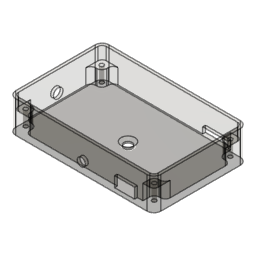
LCD Box (Autodesk Fusion 360 design; units mm, degrees)
Autodesk Fusion 360 part; units mm, degrees
sketch "Sketch1" plane through (0, 0, 0) normal (0, 1, 0) x (1, 0, 0)
  line L0 (-52.5, 33.75) -> (52.5, 33.75)
  line L1 (52.5, 33.75) -> (52.5, -33.75)
  line L2 (52.5, -33.75) -> (-52.5, -33.75)
  line L3 (-52.5, -33.75) -> (-52.5, 33.75)
  line L4 (-52.5, 33.75) -> (52.5, -33.75) construction
  dimension "d1" = 105
  dimension "d2" = 67.5
  constraint horizontal L0
  constraint vertical L1
  constraint horizontal L2
  constraint vertical L3
  constraint midpoint origin L4
  measures "d1" distance of L0.start L0.end
  measures "d2" distance of L0.start L2.end
extrude "Extrude1" add sketch "Sketch1" along normal blind 3
sketch "Sketch2" plane through (0, 3, 0) normal (0, 1, 0) x (-1, 0, 0)
  line L0 (52.5, 33.75) -> (-52.5, 33.75)
  line L1 (-52.5, 33.75) -> (-52.5, -33.75)
  line L2 (-52.5, -33.75) -> (52.5, -33.75)
  line L3 (52.5, -33.75) -> (52.5, 33.75)
  line L4 (50.5, 31.75) -> (-50.5, 31.75)
  line L5 (-50.5, 31.75) -> (-50.5, -31.75)
  line L6 (-50.5, -31.75) -> (50.5, -31.75)
  line L7 (50.5, -31.75) -> (50.5, 31.75)
  dimension "d5" = -2
extrude "Extrude2" add sketch "Sketch2" along normal blind 20
sketch "Sketch3" plane through (0, 0, -33.75) normal (0, 0, -1) x (-1, 0, 0)
  line L0 (-52.5, 0) -> (52.5, 0)
  line L1 (52.5, 0) -> (52.5, 23)
  line L2 (52.5, 23) -> (-52.5, 23)
  line L3 (-52.5, 23) -> (-52.5, 0)
  line L4 (-40.5, 7.5) -> (-22.25, 7.5)
  line L5 (-22.25, 7.5) -> (-22.25, 3)
  line L6 (-22.25, 3) -> (-40.5, 3)
  line L7 (-40.5, 3) -> (-40.5, 7.5)
  dimension "d21" = 18.25
  dimension "d22" = 4.5
  dimension "d23" = 3
  dimension "d24" = 40.5
  constraint horizontal L4
  constraint vertical L5
  constraint horizontal L6
  constraint vertical L7
  measures "d21" distance of L5.end L6.end
  measures "d22" distance of L4.start L6.end
  measures "d23" distance of origin L6
  measures "d24" distance of origin L7
extrude "Extrude3" cut sketch "Sketch3" against normal blind 3 contours L4 L5 L6 L7
sketch "Sketch4" plane through (0, 3, 0) normal (0, 1, 0) x (-1, 0, 0)
  line L0 (-22.25, -31.75) -> (50.5, -31.75)
  line L1 (50.5, -31.75) -> (50.5, 31.75)
  line L2 (50.5, 31.75) -> (-50.5, 31.75)
  line L3 (-50.5, 31.75) -> (-50.5, -31.75)
  line L4 (-50.5, -31.75) -> (-40.5, -31.75)
  line L5 (-40.5, -31.75) -> (-40.5, -33.75)
  line L6 (-40.5, -33.75) -> (-22.25, -33.75)
  line L7 (-22.25, -33.75) -> (-22.25, -31.75)
  line L8 (46.5, -27.5) -> (-46.5, -27.5) construction
  line L9 (-46.5, -27.5) -> (-46.5, 27.5) construction
  line L10 (-46.5, 27.5) -> (46.5, 27.5) construction
  line L11 (46.5, 27.5) -> (46.5, -27.5) construction
  line L12 (46.5, -27.5) -> (-46.5, 27.5) construction
  circle A0 centre (46.5, -27.5) radius 1.5
  line L13 (50.5, -23.5) -> (42.5, -23.5)
  line L14 (42.5, -23.5) -> (42.5, -31.75)
  line L15 (50.5, 0) -> (-50.5, 0) construction
  line L16 (50.5, 23.5) -> (42.5, 23.5)
  line L17 (42.5, 23.5) -> (42.5, 31.75)
  circle A1 centre (46.5, 27.5) radius 1.5
  line L18 (0, -27.5) -> (0, 27.5) construction
  line L19 (-42.5, -23.5) -> (-42.5, -31.75)
  line L20 (-50.5, -23.5) -> (-42.5, -23.5)
  circle A2 centre (-46.5, -27.5) radius 1.5
  circle A3 centre (-46.5, 27.5) radius 1.5
  line L21 (-50.5, 23.5) -> (-42.5, 23.5)
  line L22 (-42.5, 23.5) -> (-42.5, 31.75)
  dimension "d33" = 93
  dimension "d34" = 55
  dimension "d35" = 3
  dimension "d36" = 4
  dimension "d37" = 4
  constraint horizontal L8
  constraint vertical L9
  constraint horizontal L10
  constraint vertical L11
  constraint midpoint origin L12
  constraint coincident L8.start L11.end
  constraint coincident L1 L13.start
  constraint perpendicular L1 L13
  constraint coincident L0 L14.end
  constraint perpendicular L0 L14
  constraint midpoint L1 L15.start
  constraint midpoint L3 L15.end
  constraint symmetric A0 L15 A1
  constraint symmetric L13.start L15 L16.start
  constraint symmetric L13.end L15 L16.end
  constraint symmetric L14.end L15 L17.end
  constraint midpoint L8 L18.start
  constraint midpoint L10 L18.end
  constraint symmetric A0 L18 A2
  constraint symmetric L13.start L18 L20.start
  constraint symmetric L13.end L18 L19.start
  constraint symmetric L14.end L18 L19.end
  constraint symmetric L16.start L18 L21.start
  constraint symmetric L16.end L18 L21.end
  constraint symmetric L17.end L18 L22.end
  constraint symmetric A1 L18 A3
  measures "d33" distance of L8.start L8.end
  measures "d34" distance of L8.start L10.end
  measures "d35" diameter of A0
  measures "d36" distance of L8.start L13
  measures "d37" distance of L8.start L14
extrude "Extrude4" add sketch "Sketch4" along normal blind 11 contours L0 L1 L13 L14 | L1 L2 L16 L17 | L3 L4 L19 L20 | L2 L3 L21 L22
fillet "Fillet1" radius 3 4 edges at (-50.5, 18.5, -31.75) (50.5, 18.5, -31.75) (50.5, 18.5, 31.75) (-50.5, 18.5, 31.75)
fillet "Fillet2" radius 5 4 edges at (-52.5, 11.5, 33.75) (52.5, 11.5, 33.75) (52.5, 11.5, -33.75) (-52.5, 11.5, -33.75)
sketch "Sketch5" plane through (0, 0, 33.75) normal (0, 0, 1) x (1, 0, 0)
  line L0 (47.5, 0) -> (47.5, 23)
  line L1 (47.5, 23) -> (-47.5, 23)
  line L2 (-47.5, 23) -> (-47.5, 0)
  line L3 (-47.5, 0) -> (47.5, 0)
  circle A0 centre (0, 7) radius 3
  line L4 (0, 7) -> (0, 0) construction
  dimension "d58" = 6
  dimension "d59" = 7
  constraint coincident A0.centre L4.start
  constraint coincident L4.end origin
  constraint vertical L4
  measures "d58" diameter of A0
  measures "d59" distance of A0.centre L4.end
extrude "Extrude5" cut sketch "Sketch5" against normal blind 3 contours A0
sketch "Sketch6" plane through (0, 0, 33.75) normal (0, 0, 1) x (1, 0, 0)
  circle A0 centre (0, 7) radius 3
  line L0 (47.5, 0) -> (47.5, 23)
  line L1 (47.5, 23) -> (-47.5, 23)
  line L2 (-47.5, 23) -> (-47.5, 0)
  line L3 (-47.5, 0) -> (47.5, 0)
  line L4 (24, 10.5) -> (38.5, 10.5)
  line L5 (38.5, 10.5) -> (38.5, 3)
  line L6 (38.5, 3) -> (24, 3)
  line L7 (24, 3) -> (24, 10.5)
  dimension "d62" = 3
  dimension "d63" = 24
  dimension "d64" = 14.5
  dimension "d65" = 7.5
  constraint horizontal L4
  constraint vertical L5
  constraint horizontal L6
  constraint vertical L7
  measures "d62" distance of origin L6
  measures "d63" distance of origin L7
  measures "d64" distance of L4.start L4.end
  measures "d65" distance of L4.end L5.end
extrude "Extrude6" cut sketch "Sketch6" against normal blind 2 contours L4 L5 L6 L7
sketch "Sketch8" plane through (0, 3, 0) normal (0, 1, 0) x (-1, 0, 0)
  line L0 (-50.5, -23.5) -> (-42.5, -23.5)
  line L1 (-42.5, -23.5) -> (-42.5, -31.75)
  line L2 (-42.5, -31.75) -> (-40.5, -31.75)
  line L3 (-40.5, -31.75) -> (-40.5, -33.75)
  line L4 (-40.5, -33.75) -> (-22.25, -33.75)
  line L5 (-22.25, -33.75) -> (-22.25, -31.75)
  line L6 (-22.25, -31.75) -> (42.5, -31.75)
  line L7 (42.5, -31.75) -> (42.5, -23.5)
  line L8 (42.5, -23.5) -> (50.5, -23.5)
  line L9 (50.5, -23.5) -> (50.5, 23.5)
  line L10 (50.5, 23.5) -> (42.5, 23.5)
  line L11 (42.5, 23.5) -> (42.5, 31.75)
  line L12 (42.5, 31.75) -> (-24, 31.75)
  line L13 (-24, 31.75) -> (-24, 33.75)
  line L14 (-24, 33.75) -> (-38.5, 33.75)
  line L15 (-38.5, 33.75) -> (-38.5, 31.75)
  line L16 (-38.5, 31.75) -> (-42.5, 31.75)
  line L17 (-42.5, 31.75) -> (-42.5, 23.5)
  line L18 (-42.5, 23.5) -> (-50.5, 23.5)
  line L19 (-50.5, 23.5) -> (-50.5, -23.5)
  circle A0 centre (0, 0) radius 3
  dimension "d73" = 6
  constraint coincident A0.centre origin
  measures "d73" diameter of A0
extrude "Extrude8" cut sketch "Sketch8" against normal blind 6 contours A0
chamfer "Chamfer1" distance 2 angle 45 1 edges at (2.797, 3, 1.0848)
sketch "Sketch9" plane through (-52.5, 0, 0) normal (-1, 0, 0) x (0, 0, 1)
  line L0 (-28.75, 23) -> (-28.75, 0)
  line L1 (-28.75, 0) -> (28.75, 0)
  line L2 (28.75, 0) -> (28.75, 23)
  line L3 (28.75, 23) -> (-28.75, 23)
  circle A0 centre (0, 8) radius 3.5
  line L4 (0, 8) -> (0, 0) construction
  dimension "d77" = 7
  dimension "d78" = 8
  constraint coincident A0.centre L4.start
  constraint coincident L4.end origin
  constraint vertical L4
  measures "d77" diameter of A0
  measures "d78" distance of A0.centre L4.end
extrude "Extrude9" cut sketch "Sketch9" against normal blind 2 contours A0
fillet "Fillet3" radius 3.5 10 edges at (-42.5, 8.5, -23.5) (-50.5, 8.5, -23.5) (-42.5, 8.5, -31.75) (42.5, 8.5, -23.5) (50.5, 8.5, -23.5) (50.5, 8.5, 23.5) (42.5, 8.5, 23.5) (-42.5, 8.5, 31.75) (-42.5, 8.5, 23.5) (-50.5, 8.5, 23.5)
